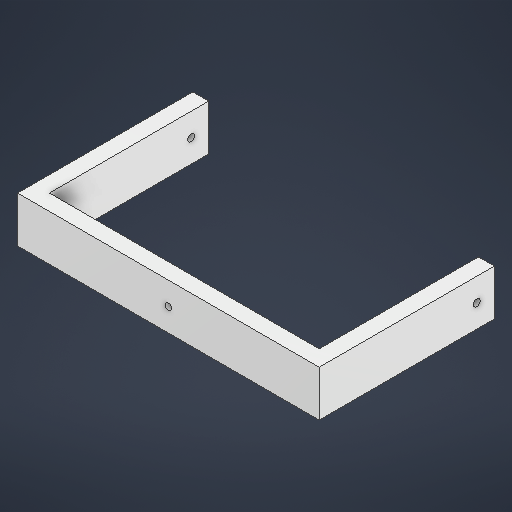
# Autodesk Inventor part: Sensor houder
Saved by Autodesk Inventor 2026.2 (Build 302298000, 298)
## iProperties
Created: 2026-05-05
Part Number: Sensor houder
Material: ABS Plastic
Document SubType Name: Modeling
Designer: Gameb
Density: 1.06 g/cm^3
Appearance: Smooth - White
Author: Gameb
Autodesk Inventor part; units mm, degrees
ref_plane "YZ Plane" through (0, 0, 0) normal (1, 0, 0) x (0, 1, 0)
ref_plane "XZ Plane" through (0, 0, 0) normal (0, 1, 0) x (-1, 0, 0)
ref_plane "XY Plane" through (0, 0, 0) normal (0, 0, 1) x (1, 0, 0)
sketch "Sketch1" plane through (0, 0, 0) normal (0, 0, 1) x (1, 0, 0)
  circle A0 centre (0, 0) radius 11.5
  circle A1 centre (0, 0) radius 1.65
  line L0 (-11.5, 0) -> (-11.5, -5)
  line L1 (-11.5, 0) -> (-11.5, 5)
  line L2 (-11.5, 5) -> (-10.3562, 5)
  line L3 (-11.5, -5) -> (-10.3562, -5)
  line L4 (11.5, 0) -> (11.5, 5)
  line L5 (11.5, 5) -> (10.3562, 5)
  line L6 (11.5, 0) -> (11.5, -5)
  line L7 (11.5, -5) -> (10.3562, -5)
  line L8 (-67.75, 0) -> (-67.75, 5)
  line L9 (-67.75, 5) -> (-11.5, 5)
  line L10 (-67.75, 0) -> (-67.75, -5)
  line L11 (-67.75, -5) -> (-11.5, -5)
  line L12 (67.75, -5) -> (67.75, 5)
  line L13 (67.75, 5) -> (11.5, 5)
  line L14 (11.5, -5) -> (67.75, -5)
  line L15 (67.75, -5) -> (71.75, -5)
  line L16 (71.75, -5) -> (71.75, 5)
  line L17 (71.75, 5) -> (67.75, 5)
  line L18 (-67.75, -5) -> (-71.75, -5)
  line L19 (-71.75, -5) -> (-71.75, 5)
  line L20 (-71.75, 5) -> (-67.75, 5)
  line L21 (0, 11.5) -> (-71.75, 11.5)
  line L22 (-71.75, 11.5) -> (-71.75, 5)
  line L23 (-71.75, -5) -> (-71.75, -11.5)
  line L24 (-71.75, -11.5) -> (0, -11.5)
  line L25 (0, -11.5) -> (71.75, -11.5)
  line L26 (71.75, -11.5) -> (71.75, -5)
  line L27 (71.75, 5) -> (71.75, 11.5)
  line L28 (0, 11.5) -> (71.75, 11.5)
  line L29 (67.75, 5) -> (67.75, 11.5)
  line L30 (67.75, 11.5) -> (63.75, 11.5)
  line L31 (63.75, 11.5) -> (63.75, -11.5)
  line L32 (-71.75, -11.5) -> (-63.75, -11.5)
  line L33 (-63.75, -11.5) -> (-63.75, 11.5)
  line L34 (-67.75, -11.5) -> (-75.75, -11.5)
  line L35 (-75.75, -11.5) -> (-75.75, 11.5)
  line L36 (-75.75, 11.5) -> (-67.75, 11.5)
  line L37 (-67.75, 11.5) -> (-67.75, -11.5)
  line L38 (67.75, 11.5) -> (75.75, 11.5)
  line L39 (75.75, 11.5) -> (75.75, -11.5)
  line L40 (75.75, -11.5) -> (67.75, -11.5)
  line L41 (67.75, -11.5) -> (67.75, 11.5)
  dimension "d0" = 23
  dimension "d1" = 3.3
  dimension "d4" = 5
  dimension "d5" = 5
  dimension "d6" = 5
  dimension "d7" = 5
  dimension "d12" = 4
  dimension "d13" = 4
  dimension "d20" = 4
  dimension "d21" = 8
  dimension "d24" = 8
  dimension "d25" = 8
  constraints: 84 end point, 18 perpendicular, 15 point on line, 7 horizontal, 6 vertical, 5 parallel, 2 coincident, 1 centre point, 1 midpoint, 10 other
  measures "d1" diameter of A1
  measures "d4" distance of L0.start L0.end
  measures "d5" distance of L0.start L1.end
  measures "d6" distance of L4.start L4.end
  measures "d7" distance of L4.start L6.end
  measures "d12" distance of L12.start L15.end
  measures "d13" distance of L10.end L18.end
  measures "d20" distance of L29.end L30.end
  measures "d21" distance of L23.end L32.end
  measures "d24" distance of L35.end L36.end
  measures "d25" distance of L39.end L40.end
extrude "Extrusion1" add sketch "Sketch1" along normal blind 8
extrude "Extrusion2" add sketch "Sketch1" against normal blind 80 contours L17 L16 L15 L12 | L29 L28 L27 L17 | L15 L26 L25 L41 | L37 L20 L22 L21 | L24 L23 L18 L37 | L27 L38 L39 L40 L26 L16 | L22 L19 L23 L34 L35 L36 | L8 L10 L18 L19 L20
sketch "Sketch4" plane through (75.75, -11.5, 8) normal (1, 0, 0) x (0, 0, -1)
  circle A0 centre (79.1099, 11.5) radius 1.75
  point P0 (8, 11.5)
  dimension "d26" = 3.5
  constraints: 1 centre point
  measures "d26" diameter of A0
extrude "Extrusion5" cut sketch "Sketch4" against normal blind 800
body "Solid1"
